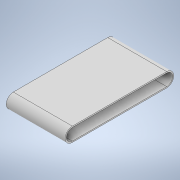
# Autodesk Inventor part: Adrian_Förderband
Saved by Autodesk Inventor 2021 (Build 250183000, 183)
## iProperties
Created: 2022-07-12
Part Number: Adrian_Förderband
Material: Generisch
Document SubType Name: Modeling
Designer: adria
Mass: 9727.88 g
Surface Area: 19844.9 cm^2
Volume: 9727.88 cm^3
Density: 1 g/cm^3
Appearance: Vorgabe
Author: adria
Autodesk Inventor part; units mm, degrees
ref_plane "YZ Plane" through (0, 0, 0) normal (1, 0, 0) x (0, 1, 0)
ref_plane "XZ Plane" through (0, 0, 0) normal (0, 1, 0) x (-1, 0, 0)
ref_plane "XY Plane" through (0, 0, 0) normal (0, 0, 1) x (1, 0, 0)
sketch "Skizze1" plane through (0, 0, 0) normal (1, 0, 0) x (0, 1, 0)
  line L0 (0, 0) -> (0, -800) construction
  line L1 (-50, 0) -> (-50, -800)
  line L2 (50, -800) -> (50, 0)
  arc A0 (50, 0) -> (-50, 0) centre (0, 0) ccw
  arc A1 (-50, -800) -> (50, -800) centre (0, -800) ccw
  line L3 (0, 0) -> (0, -800) construction
  line L4 (-60, 0) -> (-60, -800)
  line L5 (60, -800) -> (60, 0)
  arc A2 (60, 0) -> (-60, 0) centre (0, 0) ccw
  arc A3 (-60, -800) -> (60, -800) centre (0, -800) ccw
  point P0 (0, -400)
  point P1 (0, -400)
  dimension "d0" = 10
  dimension "d1" = 800
  dimension "d2" = 100
  constraints: 16 end point, 8 point on circle, 8 tangent, 4 centre point, 2 midpoint, 2 parallel, 2 vertical
  measures "d0" distance between parallel lines of L2 L5
  measures "d1" distance of L0.end L0.start
  measures "d2" distance between parallel lines of L1 L2
extrude "Extrusion1" add sketch "Skizze1" along normal mid plane 500
